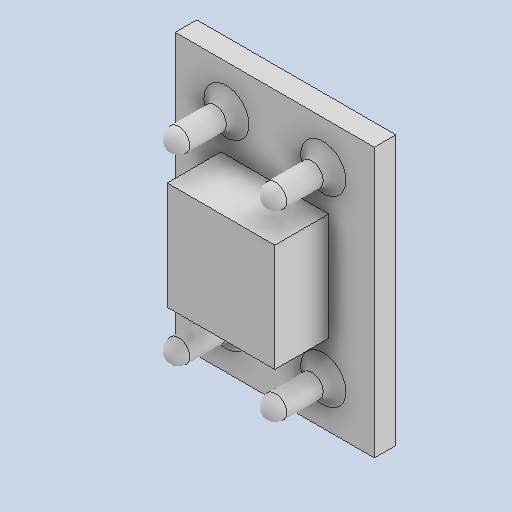
# Autodesk Inventor part: PDMS Chamber-Mold-V8 Steven
Saved by Autodesk Inventor 2022 (Build 260153000, 153)
## iProperties
Created: 2021-04-09
Part Number: PDMS Chamber-Mold-V8 Steven
Material: Generic
Document SubType Name: Modeling
Designer: Jeremy Hirota
Density: 1 g/cm^3
Appearance: Default
Author: Jeremy Hirota
Autodesk Inventor part; units mm, degrees
ref_plane "YZ Plane" through (0, 0, 0) normal (1, 0, 0) x (0, 1, 0)
ref_plane "XZ Plane" through (0, 0, 0) normal (0, 1, 0) x (-1, 0, 0)
ref_plane "XY Plane" through (0, 0, 0) normal (0, 0, 1) x (1, 0, 0)
sketch "Sketch1" plane through (0, 0, 0) normal (0, 0, 1) x (1, 0, 0)
  line L0 (-13.5, 20) -> (13.5, 20)
  line L1 (13.5, 20) -> (13.5, -20)
  line L2 (13.5, -20) -> (-13.5, -20)
  line L3 (-13.5, -20) -> (-13.5, 20)
  line L4 (-10, 10) -> (10, 10)
  line L5 (10, 10) -> (10, -10)
  line L6 (10, -10) -> (-10, -10)
  line L7 (-10, -10) -> (-10, 10)
  circle A0 centre (-8, 15) radius 2.025
  circle A1 centre (8, 15) radius 2.025
  circle A2 centre (8, -15) radius 2.025
  circle A3 centre (-8, -15) radius 2.025
  line L8 (-16.5, 23) -> (16.5, 23)
  line L9 (16.5, 23) -> (16.5, -23)
  line L10 (16.5, -23) -> (-16.5, -23)
  line L11 (-16.5, -23) -> (-16.5, 23)
  point P0 (0, 0)
  dimension "d0" = 27
  dimension "d1" = 40
  dimension "d2" = 20
  dimension "d3" = 13.5
  dimension "d4" = 20
  dimension "d5" = 20
  dimension "d6" = 3.5
  dimension "d7" = 10
  dimension "d8" = 4.05
  dimension "d9" = 5
  dimension "d10" = 5.5
  dimension "d11" = 4.05
  dimension "d12" = 5.5
  dimension "d13" = 4.05
  dimension "d14" = 5
  dimension "d15" = 4.05
  dimension "d16" = 5
  dimension "d17" = 33
  dimension "d18" = 46
  dimension "d19" = 16.5
  dimension "d20" = 23
  dimension "d29" = 5.5
  dimension "d30" = 5.5
  dimension "d31" = 5
  constraints: 24 end point, 6 parallel, 4 centre point, 3 horizontal, 3 perpendicular
  measures "d0" distance of L1.end L2.end
  measures "d1" distance of L0.end L1.end
  measures "d2" distance from line of point (0, 0) L0
  measures "d3" distance from line of L3 point (0, 0)
  measures "d4" distance of L5.end L6.end
  measures "d5" distance of L4.end L5.end
  measures "d6" distance between parallel lines of L3 L7
  measures "d7" distance between parallel lines of L0 L4
  measures "d8" diameter of A0
  measures "d9" distance from line of L0 A0.centre
  measures "d10" distance from line of L3 A0.centre
  measures "d11" diameter of A1
  measures "d12" distance from line of L1 A1.centre
  measures "d13" diameter of A2
  measures "d14" distance from line of L2 A2.centre
  measures "d15" diameter of A3
  measures "d16" distance from line of L2 A3.centre
  measures "d17" distance of L9.end L10.end
  measures "d18" distance of L8.end L9.end
  measures "d19" distance from line of point (0, 0) L11
  measures "d20" distance from line of point (0, 0) L8
  measures "d29" distance from line of L3 A3.centre
  measures "d30" distance from line of L1 A2.centre
  measures "d31" distance from line of L0 A1.centre
extrude "Extrusion1" add sketch "Sketch1" along normal blind 12 contours L4 L5 L6 L7 | A0 | A1 | A2 | A3
extrude "Extrusion2" add sketch "Sketch1" against normal blind 4 contours L0 L1 L2 L3 | L4 L5 L6 L7 | A0 | A1 | A2 | A3 | L8 L9 L10 L11
extrude "Extrusion3" add sketch "Sketch1" along normal blind 11 contours L8 L9 L10 L11
sketch "Sketch2" plane through (0, 0, 12) normal (0, 0, 1) x (1, 0, 0)
  line L0 (-10, -10) -> (10, -10) projected
  line L1 (10, -10) -> (10, 10) projected
  line L2 (10, 10) -> (-10, 10) projected
  line L3 (-10, 10) -> (-10, -10) projected
  circle A0 centre (-8, 15) radius 2.025 projected
  circle A1 centre (8, 15) radius 2.025 projected
  circle A2 centre (8, -15) radius 2.025 projected
  circle A3 centre (-8, -15) radius 2.025 projected
  point P0 (0, 0)
extrude "Extrusion4" cut sketch "Sketch2" against normal up to surface (16 mm away)
sketch "Sketch6" plane through (0, 0, -4) normal (0, 0, -1) x (-1, 0, 0)
  line L0 (-10, -10) -> (-10, 10) projected
  line L1 (10, -10) -> (-10, -10) projected
  line L2 (-10, 10) -> (10, 10)
  line L3 (10, 10) -> (10, -10)
  line L4 (10, -10) -> (-10, -10)
  line L5 (-10, -10) -> (-10, 10)
  point P0 (0, 0)
  constraints: 8 end point, 2 parallel, 1 horizontal, 1 perpendicular
extrude "Extrusion7" add sketch "Sketch6" against normal blind 14
sketch "Sketch9" plane through (0, 0, 11) normal (0, 0, 1) x (1, 0, 0)
  line L0 (-16.5, -23) -> (16.5, -23) projected
  line L1 (16.5, -23) -> (16.5, 23) projected
  line L2 (16.5, 23) -> (-16.5, 23) projected
  line L3 (-16.5, 23) -> (-16.5, -23) projected
  line L4 (-13.5, 20) -> (13.5, 20) projected
  line L5 (13.5, 20) -> (13.5, -20) projected
  line L6 (13.5, -20) -> (-13.5, -20) projected
  line L7 (-13.5, -20) -> (-13.5, 20) projected
  point P0 (0, 0)
extrude "Extrusion9" cut sketch "Sketch9" against normal blind 11
sketch "Sketch10" plane through (0, 0, -4) normal (0, 0, -1) x (-1, 0, 0)
  circle A0 centre (-8, -15) radius 2.025 projected
  circle A1 centre (8, -15) radius 2.025 projected
  circle A2 centre (-8, 15) radius 2.025 projected
  circle A3 centre (8, 15) radius 2.025 projected
  point P0 (0, 0)
extrude "Extrusion10" add sketch "Sketch10" against normal blind 4
sketch "Sketch11" plane through (0, 0, 0) normal (0, 0, 1) x (1, 0, 0)
  circle A0 centre (-9, 17) radius 2.1
  circle A1 centre (9, 17) radius 2.1
  line L0 (-16.5, -23) -> (-16.5, 23) projected
  line L1 (16.5, 23) -> (16.5, -23) projected
  line L2 (-16.5, 23) -> (16.5, 23) projected
  circle A2 centre (-9, -17) radius 2.1
  circle A3 centre (9, -17) radius 2.1
  line L3 (-16.5, -23) -> (16.5, -23)
  point P0 (0, 0)
  dimension "d70" = 4.2
  dimension "d71" = 4.2
  dimension "d72" = 7.5
  dimension "d73" = 7.5
  dimension "d74" = 6
  dimension "d75" = 6
  constraints: 4 centre point, 2 end point
  measures "d70" diameter of A0
  measures "d71" diameter of A1
  measures "d72" distance from line of A0.centre L0
  measures "d73" distance from line of A1.centre L1
  measures "d74" distance from line of L2 A1.centre
  measures "d75" distance from line of L2 A0.centre
extrude "Extrusion11" add sketch "Sketch11" along normal blind 11 contours A0 | A1 | A2 | A3
fillet "Fillet3" radius 2.1 4 edges at (-11.1, -17, 11) (6.9, -17, 11) (6.9, 17, 11) (-11.1, 17, 11)
sketch "Sketch12" plane through (0, 0, -4) normal (0, 0, -1) x (-1, 0, 0)
  line L0 (18.5, -25) -> (-18.5, -25)
  line L1 (-18.5, -25) -> (-18.5, 25)
  line L2 (-18.5, 25) -> (18.5, 25)
  line L3 (18.5, 25) -> (18.5, -25)
  line L4 (16.5, -23) -> (16.5, 23) projected
  line L5 (-16.5, -23) -> (16.5, -23) projected
  line L6 (-16.5, -23) -> (16.5, -23) projected
  line L7 (16.5, -23) -> (16.5, 23) projected
  line L8 (16.5, 23) -> (-16.5, 23) projected
  line L9 (-16.5, 23) -> (-16.5, -23) projected
  point P0 (0, 0)
  dimension "d79" = 37
  dimension "d80" = 50
  dimension "d81" = 2
  dimension "d82" = 2
  constraints: 8 end point, 2 parallel, 1 horizontal, 1 perpendicular
  measures "d79" distance of L1.end L2.end
  measures "d80" distance of L0.end L1.end
  measures "d81" distance between parallel lines of L3 L4
  measures "d82" distance between parallel lines of L0 L5
extrude "Extrusion12" add sketch "Sketch12" against normal blind 4
fillet "Fillet4" radius 2.1 4 edges at (6.9, 17, 0) (-11.1, 17, 0) (6.9, -17, 0) (-11.1, -17, 0)
body "Solid1"
